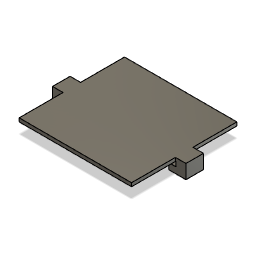
Tissue holder stage V17 (Autodesk Fusion 360 design; units mm, degrees)
Autodesk Fusion 360 part; units mm, degrees
sketch "Sketch1" plane through (0, 0, 0) normal (0, 1, 0) x (1, 0, 0) in component "Support"
  circle A0 centre (0, 0) radius 6.91
  dimension "d1" = 13.82
  constraint coincident A0.centre origin
  measures "d1" diameter of A0
extrude "Extrude1" add sketch "Sketch1" against normal blind 4 makes body 1 in component "Support"
sketch "Sketch2" plane through (0, 0, 0) normal (0, 1, 0) x (1, 0, 0) in component "Support"
  line L0 (11, -21) -> (-11, -21)
  line L1 (-11, -21) -> (-11, 21)
  line L2 (-11, 21) -> (11, 21)
  line L3 (11, 21) -> (11, -21)
  line L4 (11, -21) -> (-11, 21) construction
  line L5 (-11, -21) -> (11, 21) construction
  dimension "d4" = 22
  dimension "d5" = 42
  constraint horizontal L0
  constraint perpendicular L0 L1
  constraint parallel L0 L2
  constraint parallel L1 L3
  constraint coincident L4 origin
  constraint coincident L5 origin
  measures "d4" distance of L1.end L2.end
  measures "d5" distance of L0.end L1.end
extrude "Extrude2" add sketch "Sketch2" along normal blind 1 bodies 1 in component "Support"
ref_plane "WorkPlane1" through (0, 1, 0) normal (0, 1, 0) x (0, 0, 1) in component "Stage"
sketch "Sketch1 (2)" plane through (0, 1, 0) normal (0, 1, 0) x (1, 0, 0) in component "Stage"
  line L0 (19, -15) -> (-19, -15)
  line L1 (-19, -15) -> (-19, 15)
  line L2 (-19, 15) -> (19, 15)
  line L3 (19, 15) -> (19, -15)
  line L4 (19, -15) -> (-19, 15) construction
  line L5 (-19, -15) -> (19, 15) construction
  dimension "d9" = 38
  dimension "d10" = 30
  constraint horizontal L0
  constraint perpendicular L0 L1
  constraint parallel L0 L2
  constraint parallel L1 L3
  constraint coincident L4 origin
  constraint coincident L5 origin
  measures "d9" distance of L1.end L2.end
  measures "d10" distance of L0.end L1.end
extrude "Extrude1'" add sketch "Sketch1 (2)" along normal blind 1 separate body makes body 2 in component "Stage"
sketch "Sketch2 (2)" plane through (0, 1, 0) normal (0, -1, 0) x (1, 0, 0) in component "Stage"
  line L0 (-19, -15) -> (19, -15)
  line L1 (19, -15) -> (19, 15)
  line L2 (19, 15) -> (-19, 15)
  line L3 (-19, 15) -> (-19, -15)
  line L4 (19, 15) -> (16.12, 15)
  line L5 (16.12, 15) -> (16.12, -15)
  line L6 (16.12, -15) -> (19, -15)
  line L7 (19, -15) -> (19, 15)
  line L8 (16.12, -15) -> (19, -15)
  line L9 (19, -15) -> (19, -10)
  line L10 (19, -10) -> (16.12, -10)
  line L11 (16.12, -10) -> (16.12, -15)
  dimension "d13" = 2.88
  dimension "d14" = 30
  dimension "d72" = 5
  constraint horizontal L4
  constraint vertical L5
  constraint horizontal L6
  constraint vertical L7
  constraint coincident L1.end L2.start
  constraint horizontal L8
  constraint vertical L9
  constraint horizontal L10
  constraint vertical L11
  measures "d13" distance of L1.end L4.end
  measures "d14" distance of L1.end L0.end
  measures "d72" distance of L5.end L10.end
extrude "Extrude2'" add sketch "Sketch2 (2)" along normal blind 3 contours L0 L1 L5 L6 L7 L8 L9 L10 L11 | L1 L2 L4 L5 L7 L10 bodies 2 in component "Stage"
sketch "Sketch3" plane through (16.12, 0, 0) normal (-1, 0, 0) x (0, 0, 1) in component "Stage"
  line L0 (15, 1) -> (-15, 1)
  line L1 (-15, 1) -> (-15, -2)
  line L2 (-15, -2) -> (15, -2)
  line L3 (15, -2) -> (15, 1)
  line L4 (-15, -2) -> (15, -2)
  line L5 (15, -2) -> (15, -0.05)
  line L6 (15, -0.05) -> (-15, -0.05)
  line L7 (-15, -0.05) -> (-15, -2)
  dimension "d17" = 30
  dimension "d18" = 1.95
  constraint horizontal L4
  constraint vertical L5
  constraint horizontal L6
  constraint vertical L7
  constraint coincident L1.end L2.start
  measures "d17" distance of L1.end L2.end
  measures "d18" distance of L1.end L6.end
extrude "Extrude3" add sketch "Sketch3" along normal blind 1.5 contours L1 L2 L3 L4 L5 L6 L7 bodies 2 in component "Stage"
sketch "Sketch4" plane through (0, 1, 0) normal (0, -1, 0) x (1, 0, 0) in component "Stage"
  line L0 (16.12, -15) -> (16.12, 15)
  line L1 (16.12, 15) -> (-19, 15)
  line L2 (-19, 15) -> (-19, -15)
  line L3 (-19, -15) -> (16.12, -15)
  line L4 (-19, 15) -> (-16.12, 15)
  line L5 (-16.12, 15) -> (-16.12, -15)
  line L6 (-16.12, -15) -> (-19, -15)
  line L7 (-19, -15) -> (-19, 15)
  line L8 (-19, 15) -> (-16.18, 15)
  line L9 (-16.18, 15) -> (-16.18, 10)
  line L10 (-16.18, 10) -> (-19, 10)
  line L11 (-19, 10) -> (-19, 15)
  dimension "d21" = 2.88
  dimension "d22" = 30
  dimension "d73" = 5
  constraint horizontal L4
  constraint vertical L5
  constraint horizontal L6
  constraint vertical L7
  constraint coincident L1.end L2.start
  constraint horizontal L8
  constraint vertical L9
  constraint horizontal L10
  constraint vertical L11
  measures "d21" distance of L1.end L4.end
  measures "d22" distance of L1.end L2.end
  measures "d73" distance of L1.end L10.end
extrude "Extrude4" add sketch "Sketch4" along normal blind 3 contours L1 L2 L3 L4 L5 L6 L7 L9 L10 | L1 L2 L4 L7 L8 L9 L10 L11 bodies 2 in component "Stage"
sketch "Sketch5" plane through (-16.12, 0, 0) normal (1, 0, 0) x (0, 0, -1) in component "Stage"
  line L0 (15, 1) -> (-15, 1)
  line L1 (-15, 1) -> (-15, -2)
  line L2 (-15, -2) -> (15, -2)
  line L3 (15, -2) -> (15, 1)
  line L4 (-15, -2) -> (15, -2)
  line L5 (15, -2) -> (15, -0.05)
  line L6 (15, -0.05) -> (-15, -0.05)
  line L7 (-15, -0.05) -> (-15, -2)
  dimension "d25" = 30
  dimension "d26" = 1.95
  constraint horizontal L4
  constraint vertical L5
  constraint horizontal L6
  constraint vertical L7
  constraint coincident L1.end L2.start
  measures "d25" distance of L1.end L2.end
  measures "d26" distance of L1.end L6.end
extrude "Extrude5" add sketch "Sketch5" along normal blind 1.5 contours L1 L2 L3 L4 L5 L6 L7 bodies 2 in component "Stage"
extrude "Extrude6" cut 1 faces at (-16.12, 0.65, -5) along direction (-1, 0, 0) blind 0.1 on bodies 2 bodies 2 in component "Stage"
extrude "Extrude7" cut 1 faces at (16.12, 0.65, -5) along direction (1, 0, 0) blind 0.1 on bodies 2 bodies 2 in component "Stage"
extrude "Extrude8" cut 1 faces at (-15.1533, -0.05, -5) along direction (0, -1, 0) blind 0.15 on bodies 2 bodies 2 in component "Stage"
extrude "Extrude9" cut 1 faces at (15.6867, -0.05, 5) along direction (0, -1, 0) blind 0.15 on bodies 2 bodies 2 in component "Stage"
sketch "Sketch1 (3)" plane through (0, 0, 0) normal (0, 1, 0) x (1, 0, 0) in component "Holder"
  circle A0 centre (0, 0) radius 7
  line L0 (7.5251, -10) -> (-10, -10)
  line L1 (-10, -10) -> (-10, 7.5251)
  line L2 (-7.5251, 10) -> (10, 10)
  line L3 (10, 10) -> (10, -7.5251)
  line L4 (22.0971, -19.6222) -> (19.6222, -22.0971)
  line L5 (-22.0971, 19.6222) -> (-19.6222, 22.0971)
  line L6 (10, -7.5251) -> (22.0971, -19.6222)
  line L7 (19.6222, -22.0971) -> (7.5251, -10)
  line L8 (-19.6222, 22.0971) -> (-7.5251, 10)
  line L9 (-10, 7.5251) -> (-22.0971, 19.6222)
  dimension "d41" = 14
  dimension "d44" = 3.5
  dimension "d45" = 59
  constraint coincident A0.centre origin
  constraint horizontal L0
  constraint perpendicular L0 L1
  constraint parallel L0 L2
  constraint parallel L1 L3
  constraint perpendicular L4 L7
  constraint parallel L4 L5
  constraint parallel L7 L8
  constraint coincident L3.end L8
  constraint collinear L6 L8
  measures "d41" diameter of A0
  measures "d44" distance of L5.start L5.end
  measures "d45" distance of L4.end L5.start
extrude "Extrude1''" add sketch "Sketch1 (3)" along normal blind 4 separate body makes body 3 in component "Holder"
sketch "Sketch2 (3)" plane through (0, 4, 0) normal (0, 1, 0) x (-1, 0, 0) in component "Holder"
  circle A0 centre (0, 0) radius 7
  line L0 (10, -7.5251) -> (10, 10)
  line L1 (10, 10) -> (-7.5251, 10)
  line L2 (-7.5251, 10) -> (-19.6222, 22.0971)
  line L3 (-19.6222, 22.0971) -> (-22.0971, 19.6222)
  line L4 (-22.0971, 19.6222) -> (-10, 7.5251)
  line L5 (-10, 7.5251) -> (-10, -10)
  line L6 (-10, -10) -> (7.5251, -10)
  line L7 (7.5251, -10) -> (19.6222, -22.0971)
  line L8 (19.6222, -22.0971) -> (22.0971, -19.6222)
  line L9 (22.0971, -19.6222) -> (10, -7.5251)
  line L10 (20.8597, -20.8597) -> (18.7383, -18.7383)
  line L11 (18.7383, -18.7383, 0) -> (32.1734, -32.1734, 32.909)
  line L12 (20.8597, -20.8597, 0) -> (20.8597, -20.8597, 2)
  line L13 (20.8597, -20.8597, 2) -> (34.2947, -34.2947, 34.909)
  line L14 (32.1734, -32.1734, 32.909) -> (33.4597, -33.4597, 32.8636)
  dimension "d55" = 38
  dimension "d56" = 2
  dimension "d57" = 38
ref_plane "WorkPlane1" through (0, 12.125, 0) normal (0.707107, 0, 0.707107) x (0, 1, 0) in component "Holder"
extrude "Extrude2''" add sketch "Sketch2 (3)" along normal mid plane 3.5 separate body contours L10 L11 L12 L13 L14 in plane through (0, 4, 0) normal (-0.707107, 0, 0.707107) makes body 4 in component "Holder"
mirror "Mirror1" about plane through (0, 12.125, 0) normal (0.707107, 0, 0.707107) of bodies 4 makes body 5 in component "Holder"
combine "Combine1" operation add target body 3 tool bodies 4 5 in component "Holder"
extrude "Extrude3'" add 1 faces at (-11, 0.3333, 7) along direction (-1, 0, 0) blind 5 on bodies 1 bodies 1 in component "Support"
extrude "Extrude4'" add 1 faces at (11, 0.3333, -7) along direction (1, 0, 0) blind 5 on bodies 1 bodies 1 in component "Support"
sketch "Sketch3 (2)" plane through (0, 0, 0) normal (0, -1, 0) x (1, 0, 0) in component "Support"
  line L0 (-16, -21) -> (16, -21)
  line L1 (16, -21) -> (16, 21)
  line L2 (16, 21) -> (-16, 21)
  line L3 (-16, 21) -> (-16, -21)
  circle A0 centre (0, 0) radius 6.91
  line L4 (11, -10) -> (12, -10)
  line L5 (12, -10) -> (12, 5)
  line L6 (12, 5) -> (11, 5)
  line L7 (11, 5) -> (11, -10)
  line L8 (-11, 10) -> (-12, 10)
  line L9 (-12, 10) -> (-12, -5)
  line L10 (-12, -5) -> (-11, -5)
  line L11 (-11, -5) -> (-11, 10)
  dimension "d67" = 15
  constraint horizontal L4
  constraint vertical L5
  constraint horizontal L6
  constraint vertical L7
  constraint horizontal L8
  constraint vertical L9
  constraint horizontal L10
  constraint vertical L11
  measures "d67" distance of L4.start L6.end
extrude "Extrude5'" add sketch "Sketch3 (2)" along normal blind 1 separate body contours L4 L5 L6 L7 makes body 6 in component "Support"
extrude "Extrude6'" add sketch "Sketch3 (2)" along normal blind 1 separate body contours L8 L9 L10 L11 makes body 7 in component "Support"
combine "Combine1'" operation add target body 1 tool bodies 6 7 in component "Support"
delete_body "RemoveBody1" bodies 2 in component "Stage"
extrude "Extrude10" add sketch "Sketch1 (2)" along normal blind 1 separate body makes body 8 in component "Stage"
extrude "Extrude11" add sketch "Sketch4" sketch "Sketch2 (2)" along normal blind 3 contours L1 L2 L4 L7 L8 L9 L10 L11 of sketch 2 contours L0 L1 L5 L6 L7 L8 L9 L10 L11 bodies 8 in component "Stage"
sketch "Sketch6" plane through (-16.18, 0, 0) normal (1, 0, 0) x (0, 0, -1) in component "Stage"
  line L0 (-10, 1) -> (-15, 1)
  line L1 (-15, 1) -> (-15, -2)
  line L2 (-15, -2) -> (-10, -2)
  line L3 (-10, -2) -> (-10, 1)
  line L4 (-15, -2) -> (-10, -2)
  line L5 (-10, -2) -> (-10, -0.24)
  line L6 (-10, -0.24) -> (-15, -0.24)
  line L7 (-15, -0.24) -> (-15, -2)
  dimension "d78" = 5
  dimension "d79" = 1.76
  constraint horizontal L4
  constraint vertical L5
  constraint horizontal L6
  constraint vertical L7
  constraint coincident L1.end L2.start
  measures "d78" distance of L1.end L2.end
  measures "d79" distance of L1.end L6.end
sketch "Sketch7" plane through (16.12, 0, 0) normal (-1, 0, 0) x (0, 0, 1) in component "Stage"
  line L0 (-10, 1) -> (-15, 1)
  line L1 (-15, 1) -> (-15, -2)
  line L2 (-15, -2) -> (-10, -2)
  line L3 (-10, -2) -> (-10, 1)
  line L4 (-15, -2) -> (-10, -2)
  line L5 (-10, -2) -> (-10, -0.24)
  line L6 (-10, -0.24) -> (-15, -0.24)
  line L7 (-15, -0.24) -> (-15, -2)
  dimension "d80" = 5
  dimension "d81" = 1.76
  constraint horizontal L4
  constraint vertical L5
  constraint horizontal L6
  constraint vertical L7
  constraint coincident L1.end L2.start
  measures "d80" distance of L1.end L2.end
  measures "d81" distance of L1.end L6.end
extrude "Extrude12" add sketch "Sketch7" along normal blind 2 contours L1 L2 L3 L4 L5 L6 L7 bodies 8 in component "Stage"
extrude "Extrude13" add sketch "Sketch6" along normal blind 2 contours L1 L2 L3 L4 L5 L6 L7 bodies 8 in component "Stage"
sketch "Sketch8" plane through (0, 1, 0) normal (0, -1, 0) x (1, 0, 0) in component "Stage"
  line L0 (16.12, -15) -> (16.12, -10)
  line L1 (16.12, -10) -> (19, -10)
  line L2 (19, -10) -> (19, 15)
  line L3 (19, 15) -> (-16.18, 15)
  line L4 (-16.18, 15) -> (-16.18, 10)
  line L5 (-16.18, 10) -> (-19, 10)
  line L6 (-19, 10) -> (-19, -15)
  line L7 (-19, -15) -> (16.12, -15)
sketch "Sketch9" plane through (0, 1, 0) normal (0, -1, 0) x (1, 0, 0) in component "Stage"
  line L0 (19, 15) -> (16, 15)
  line L1 (16, 15) -> (16, -10)
  line L2 (16, -10) -> (19, -10)
  line L3 (19, -10) -> (19, 15)
  line L4 (-19, -15) -> (-16, -15)
  line L5 (-16, -15) -> (-16, 10)
  line L6 (-16, 10) -> (-19, 10)
  line L7 (-19, 10) -> (-19, -15)
  constraint horizontal L0
  constraint vertical L1
  constraint horizontal L2
  constraint vertical L3
  constraint horizontal L4
  constraint vertical L5
  constraint horizontal L6
  constraint vertical L7
extrude "Extrude14" cut sketch "Sketch9" against normal blind 1 bodies 8 in component "Stage"
sketch "Sketch4 (2)" plane through (0, 1, 0) normal (0, 1, 0) x (-1, 0, 0) in component "Support"
  line L0 (-16, -21) -> (16, -21)
  line L1 (16, -21) -> (16, 21)
  line L2 (16, 21) -> (-16, 21)
  line L3 (-16, 21) -> (-16, -21)
  line L4 (11.0067, 21) -> (9.0067, 21)
  line L5 (9.0067, 21) -> (9.0067, 20)
  line L6 (9.0067, 20) -> (11.0067, 20)
  line L7 (11.0067, 20) -> (11.0067, 21)
  line L8 (9.0067, 15) -> (11.0067, 15)
  line L9 (9.0067, 16) -> (9.0067, 15)
  line L10 (11.0067, 16) -> (9.0067, 16)
  line L11 (11.0067, 15) -> (11.0067, 16)
  line L12 (9.0067, 5) -> (11.0067, 5)
  line L13 (9.0067, 6) -> (9.0067, 5)
  line L14 (11.0067, 6) -> (9.0067, 6)
  line L15 (11.0067, 5) -> (11.0067, 6)
  line L16 (9.0067, 10) -> (11.0067, 10)
  line L17 (9.0067, 11) -> (9.0067, 10)
  line L18 (11.0067, 11) -> (9.0067, 11)
  line L19 (11.0067, 10) -> (11.0067, 11)
  line L20 (11.0067, 1) -> (9.0067, 1)
  line L21 (9.0067, 0) -> (11.0067, 0)
  line L22 (9.0067, 1) -> (9.0067, 0)
  line L23 (11.0067, 0) -> (11.0067, 1)
  line L24 (11.0067, -4) -> (9.0067, -4)
  line L25 (9.0067, -4) -> (9.0067, -5)
  line L26 (11.0067, -5) -> (11.0067, -4)
  line L27 (9.0067, -5) -> (11.0067, -5)
  line L28 (11.0067, -9) -> (9.0067, -9)
  line L29 (9.0067, -10) -> (11.0067, -10)
  line L30 (11.0067, -10) -> (11.0067, -9)
  line L31 (9.0067, -9) -> (9.0067, -10)
  line L32 (11.0067, -14) -> (9.0067, -14)
  line L33 (9.0067, -14) -> (9.0067, -15)
  line L34 (9.0067, -15) -> (11.0067, -15)
  line L35 (11.0067, -15) -> (11.0067, -14)
  line L36 (11.0067, -19) -> (9.0067, -19)
  line L37 (9.0067, -20) -> (11.0067, -20)
  line L38 (11.0067, -20) -> (11.0067, -19)
  line L39 (9.0067, -19) -> (9.0067, -20)
  line L40 (-10.9933, 21) -> (-10.9933, 20)
  line L41 (-10.9933, 20) -> (-8.9933, 20)
  line L42 (-8.9933, 20) -> (-8.9933, 21)
  line L43 (-8.9933, 21) -> (-10.9933, 21)
  line L44 (-10.9933, 16) -> (-10.9933, 15)
  line L45 (-10.9933, 15) -> (-8.9933, 15)
  line L46 (-8.9933, 16) -> (-10.9933, 16)
  line L47 (-8.9933, 15) -> (-8.9933, 16)
  line L48 (-10.9933, 10) -> (-8.9933, 10)
  line L49 (-8.9933, 11) -> (-10.9933, 11)
  line L50 (-10.9933, 11) -> (-10.9933, 10)
  line L51 (-8.9933, 10) -> (-8.9933, 11)
  line L52 (-10.9933, 6) -> (-10.9933, 5)
  line L53 (-8.9933, 6) -> (-10.9933, 6)
  line L54 (-10.9933, 5) -> (-8.9933, 5)
  line L55 (-8.9933, 5) -> (-8.9933, 6)
  line L56 (-8.9933, 0) -> (-8.9933, 1)
  line L57 (-10.9933, 0) -> (-8.9933, 0)
  line L58 (-8.9933, 1) -> (-10.9933, 1)
  line L59 (-10.9933, 1) -> (-10.9933, 0)
  line L60 (-8.9933, -4) -> (-10.9933, -4)
  line L61 (-10.9933, -4) -> (-10.9933, -5)
  line L62 (-10.9933, -5) -> (-8.9933, -5)
  line L63 (-8.9933, -5) -> (-8.9933, -4)
  line L64 (-8.9933, -9) -> (-10.9933, -9)
  line L65 (-10.9933, -10) -> (-8.9933, -10)
  line L66 (-10.9933, -9) -> (-10.9933, -10)
  line L67 (-8.9933, -10) -> (-8.9933, -9)
  line L68 (-8.9933, -14) -> (-10.9933, -14)
  line L69 (-10.9933, -14) -> (-10.9933, -15)
  line L70 (-8.9933, -15) -> (-8.9933, -14)
  line L71 (-10.9933, -15) -> (-8.9933, -15)
  line L72 (-8.9933, -19) -> (-10.9933, -19)
  line L73 (-10.9933, -19) -> (-10.9933, -20)
  line L74 (-10.9933, -20) -> (-8.9933, -20)
  line L75 (-8.9933, -20) -> (-8.9933, -19)
  dimension "d88" = 2
  dimension "d89" = 1
  dimension "d90" = 2
  dimension "d91" = 1
  dimension "d92" = 2
  dimension "d93" = 1
  dimension "d94" = 2
  dimension "d95" = 1
  dimension "d96" = 2
  dimension "d97" = 1
  dimension "d98" = 2
  dimension "d99" = 1
  dimension "d100" = 2
  dimension "d101" = 1
  dimension "d102" = 2
  dimension "d103" = 1
  dimension "d104" = 2
  dimension "d105" = 1
  dimension "d106" = 2
  dimension "d107" = 1
  dimension "d108" = 2
  dimension "d109" = 1
  dimension "d110" = 2
  dimension "d111" = 1
  dimension "d112" = 2
  dimension "d113" = 1
  dimension "d114" = 2
  dimension "d115" = 1
  dimension "d116" = 2
  dimension "d117" = 1
  dimension "d118" = 2
  dimension "d119" = 1
  dimension "d120" = 2
  dimension "d121" = 1
  dimension "d122" = 2
  dimension "d123" = 1
  constraint horizontal L4
  constraint vertical L5
  constraint horizontal L6
  constraint vertical L7
  constraint coincident L2 L4.start
  constraint horizontal L10
  constraint vertical L9
  constraint horizontal L8
  constraint vertical L11
  constraint horizontal L18
  constraint vertical L17
  constraint horizontal L16
  constraint vertical L19
  constraint horizontal L14
  constraint vertical L13
  constraint horizontal L12
  constraint vertical L15
  constraint horizontal L20
  constraint vertical L22
  constraint horizontal L21
  constraint vertical L23
  constraint horizontal L24
  constraint vertical L25
  constraint horizontal L27
  constraint vertical L26
  constraint horizontal L28
  constraint vertical L31
  constraint horizontal L29
  constraint vertical L30
  constraint horizontal L32
  constraint vertical L33
  constraint horizontal L34
  constraint vertical L35
  constraint horizontal L36
  constraint vertical L39
  constraint horizontal L37
  constraint vertical L38
  constraint horizontal L43
  constraint vertical L40
  constraint horizontal L41
  constraint vertical L42
  constraint horizontal L46
  constraint vertical L44
  constraint horizontal L45
  constraint vertical L47
  constraint horizontal L49
  constraint vertical L50
  constraint horizontal L48
  constraint vertical L51
  constraint horizontal L53
  constraint vertical L52
  constraint horizontal L54
  constraint vertical L55
  constraint horizontal L58
  constraint vertical L59
  constraint horizontal L57
  constraint vertical L56
  constraint horizontal L60
  constraint vertical L61
  constraint horizontal L62
  constraint vertical L63
  constraint horizontal L64
  constraint vertical L66
  constraint horizontal L65
  constraint vertical L67
  constraint horizontal L68
  constraint vertical L69
  constraint horizontal L71
  constraint vertical L70
  constraint horizontal L72
  constraint vertical L73
  constraint horizontal L74
  constraint vertical L75
  measures "d88" distance of L4.start L4.end
  measures "d89" distance of L4.start L6.end
  measures "d90" distance of L9.start L10.start
  measures "d91" distance of L8.end L10.start
  measures "d92" distance of L17.start L18.start
  measures "d93" distance of L16.end L18.start
  measures "d94" distance of L14.start L13.start
  measures "d95" distance of L12.end L14.start
  measures "d96" distance of L20.end L20.start
  measures "d97" distance of L21.end L20.start
  measures "d98" distance of L24.start L24.end
  measures "d99" distance of L26.start L24.start
  measures "d100" distance of L28.end L28.start
  measures "d101" distance of L29.end L28.start
  measures "d102" distance of L32.end L32.start
  measures "d103" distance of L34.end L32.start
  measures "d104" distance of L36.start L36.end
  measures "d105" distance of L37.end L36.start
  measures "d106" distance of L40.start L42.end
  measures "d107" distance of L41.end L42.end
  measures "d108" distance of L46.start L44.start
  measures "d109" distance of L45.end L46.start
  measures "d110" distance of L49.end L49.start
  measures "d111" distance of L48.end L49.start
  measures "d112" distance of L52.start L53.start
  measures "d113" distance of L54.end L53.start
  measures "d114" distance of L56.end L58.end
  measures "d115" distance of L56.start L56.end
  measures "d116" distance of L60.start L60.end
  measures "d117" distance of L60.start L62.end
  measures "d118" distance of L64.start L64.end
  measures "d119" distance of L65.end L64.start
  measures "d120" distance of L68.start L68.end
  measures "d121" distance of L70.start L68.start
  measures "d122" distance of L72.start L72.end
  measures "d123" distance of L72.start L74.end
extrude "Extrude7'" cut sketch "Sketch4 (2)" against normal blind 1 contours L2 L40 L41 L42 L43 | L2 L4 L5 L6 L7 | L8 L9 L10 L11 | L12 L13 L14 L15 | L16 L17 L18 L19 | L20 L21 L22 L23 | L24 L25 L26 L27 | L28 L29 L30 L31 | L32 L33 L34 L35 | L36 L37 L38 L39 | L44 L45 L46 L47 | L48 L49 L50 L51 | L52 L53 L54 L55 | L56 L57 L58 L59 | L60 L61 L62 L63 | L64 L65 L66 L67 | L68 L69 L70 L71 | L72 L73 L74 L75 bodies 1 in component "Support"
delete_body "RemoveBody2" bodies 8 in component "Stage"
extrude "Extrude15" add sketch "Sketch1 (2)" along normal blind 1 separate body makes body 9 in component "Stage"
sketch "Sketch10" plane through (0, 1, 0) normal (0, -1, 0) x (1, 0, 0) in component "Stage"
  line L0 (-19, -15) -> (19, -15)
  line L1 (19, -15) -> (19, 15)
  line L2 (19, 15) -> (-19, 15)
  line L3 (-19, 15) -> (-19, -15)
  line L4 (-19, -15) -> (-16, -15)
  line L5 (-16, -15) -> (-16, -2.5)
  line L6 (-16, -2.5) -> (-19, -2.5)
  line L7 (-19, -2.5) -> (-19, -15)
  line L8 (-19, 15) -> (-16, 15)
  line L9 (-16, 15) -> (-16, 2.5)
  line L10 (-16, 2.5) -> (-19, 2.5)
  line L11 (-19, 2.5) -> (-19, 15)
  line L12 (19, 15) -> (16, 15)
  line L13 (16, 15) -> (16, 2.5)
  line L14 (16, 2.5) -> (19, 2.5)
  line L15 (19, 2.5) -> (19, 15)
  line L16 (19, -15) -> (16, -15)
  line L17 (16, -15) -> (16, -2.5)
  line L18 (16, -2.5) -> (19, -2.5)
  line L19 (19, -2.5) -> (19, -15)
  dimension "d135" = 3
  dimension "d136" = 12.5
  dimension "d137" = 3
  dimension "d138" = 12.5
  dimension "d139" = 3
  dimension "d140" = 12.5
  dimension "d141" = 3
  dimension "d142" = 12.5
  constraint horizontal L4
  constraint vertical L5
  constraint horizontal L6
  constraint vertical L7
  constraint coincident L0.start L3.end
  constraint horizontal L8
  constraint vertical L9
  constraint horizontal L10
  constraint vertical L11
  constraint coincident L2.end L3.start
  constraint horizontal L12
  constraint vertical L13
  constraint horizontal L14
  constraint vertical L15
  constraint coincident L1.end L2.start
  constraint horizontal L16
  constraint vertical L17
  constraint horizontal L18
  constraint vertical L19
  constraint coincident L0.end L1.start
  measures "d135" distance of L0.start L4.end
  measures "d136" distance of L0.start L6.end
  measures "d137" distance of L2.end L8.end
  measures "d138" distance of L2.end L10.end
  measures "d139" distance of L1.end L12.end
  measures "d140" distance of L1.end L14.end
  measures "d141" distance of L0.end L16.end
  measures "d142" distance of L0.end L18.end
extrude "Extrude16" cut sketch "Sketch10" against normal blind 1 contours L0 L3 L4 L5 L6 L7 | L0 L1 L16 L17 L18 L19 | L2 L3 L8 L9 L10 L11 | L1 L2 L12 L13 L14 L15 bodies 9 in component "Stage"
sketch "Sketch11" plane through (0, 1, 0) normal (0, -1, 0) x (1, 0, 0) in component "Stage"
  line L0 (19, -2.5) -> (16.12, -2.5)
  line L1 (16.12, -2.5) -> (16.12, 2.5)
  line L2 (16.12, 2.5) -> (19, 2.5)
  line L3 (19, 2.5) -> (19, -2.5)
  line L4 (-19, -2.5) -> (-16.12, -2.5)
  line L5 (-16.12, -2.5) -> (-16.12, 2.5)
  line L6 (-16.12, 2.5) -> (-19, 2.5)
  line L7 (-19, 2.5) -> (-19, -2.5)
  dimension "d145" = 2.88
  dimension "d146" = 5
  dimension "d147" = 2.88
  dimension "d148" = 5
  constraint horizontal L0
  constraint vertical L1
  constraint horizontal L2
  constraint vertical L3
  constraint horizontal L4
  constraint vertical L5
  constraint horizontal L6
  constraint vertical L7
  measures "d145" distance of L0.start L0.end
  measures "d146" distance of L0.start L2.end
  measures "d147" distance of L4.start L4.end
  measures "d148" distance of L4.start L6.end
extrude "Extrude17" add sketch "Sketch11" along normal blind 3 bodies 9 in component "Stage"
sketch "Sketch12" plane through (-16.12, 0, 0) normal (1, 0, 0) x (0, 0, -1) in component "Stage"
  line L0 (2.5, 1) -> (-2.5, 1)
  line L1 (-2.5, 1) -> (-2.5, -2)
  line L2 (-2.5, -2) -> (2.5, -2)
  line L3 (2.5, -2) -> (2.5, 1)
  line L4 (-2.5, -2) -> (2.5, -2)
  line L5 (2.5, -2) -> (2.5, -0.24)
  line L6 (2.5, -0.24) -> (-2.5, -0.24)
  line L7 (-2.5, -0.24) -> (-2.5, -2)
  dimension "d151" = 5
  dimension "d152" = 1.76
  constraint horizontal L4
  constraint vertical L5
  constraint horizontal L6
  constraint vertical L7
  constraint coincident L1.end L2.start
  measures "d151" distance of L1.end L2.end
  measures "d152" distance of L1.end L6.end
extrude "Extrude18" add sketch "Sketch12" along normal blind 2 contours L1 L2 L3 L4 L5 L6 L7 bodies 9 in component "Stage"
sketch "Sketch13" plane through (16.12, 0, 0) normal (-1, 0, 0) x (0, 0, 1) in component "Stage"
  line L0 (2.5, 1) -> (-2.5, 1)
  line L1 (-2.5, 1) -> (-2.5, -2)
  line L2 (-2.5, -2) -> (2.5, -2)
  line L3 (2.5, -2) -> (2.5, 1)
  line L4 (-2.5, -2) -> (2.5, -2)
  line L5 (2.5, -2) -> (2.5, -0.24)
  line L6 (2.5, -0.24) -> (-2.5, -0.24)
  line L7 (-2.5, -0.24) -> (-2.5, -2)
  dimension "d155" = 5
  dimension "d156" = 1.76
  constraint horizontal L4
  constraint vertical L5
  constraint horizontal L6
  constraint vertical L7
  constraint coincident L1.end L2.start
  measures "d155" distance of L1.end L2.end
  measures "d156" distance of L1.end L6.end
extrude "Extrude19" add sketch "Sketch13" along normal blind 2 contours L1 L2 L3 L4 L5 L6 L7 bodies 9 in component "Stage"
component "Support" placed x (1, 0, 0) y (0, 1, 0) z (0, 0, 1) at (0, 0, 0)
component "Stage" placed x (1, 0, 0) y (0, 1, 0) z (0, 0, 1) at (0, 0, -1)
component "Holder" placed x (1, 0, 0) y (0, 1, 0) z (0, 0, 1) at (0, -4, 0)
